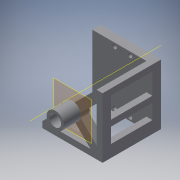
# Autodesk Inventor part: Sy_holder
Saved by Autodesk Inventor 2018 (Build 220112000, 112)
## iProperties
Created: 2018-10-01
Part Number: Sy_holder
Material: Generic
Document SubType Name: Modeling
Designer: David
Density: 1 g/cm^3
Appearance: Default
Author: David
Autodesk Inventor part; units mm, degrees
ref_plane "YZ Plane" through (0, 0, 0) normal (1, 0, 0) x (0, 1, 0)
ref_plane "XZ Plane" through (0, 0, 0) normal (0, 1, 0) x (-1, 0, 0)
ref_plane "XY Plane" through (0, 0, 0) normal (0, 0, 1) x (1, 0, 0)
sketch "Sketch1" plane through (0, 0, 0) normal (0, 1, 0) x (-1, 0, 0)
  line L0 (-17.5, -17.5) -> (17.5, -17.5)
  line L1 (17.5, -17.5) -> (17.5, 17.5)
  line L2 (17.5, 17.5) -> (-17.5, 17.5)
  line L3 (-17.5, 17.5) -> (-17.5, -17.5)
  line L4 (-17.5, -17.5) -> (17.5, 17.5) construction
  line L5 (17.5, -17.5) -> (-17.5, 17.5) construction
  point P0 (0, 0)
  dimension "d0" = 35
  dimension "d1" = 35
  constraints: 12 end point, 2 midpoint, 2 parallel, 1 horizontal, 1 perpendicular
  measures "d0" distance of L2.end L1.end
  measures "d1" distance of L1.end L0.end
extrude "Extrusion1" add sketch "Sketch1" along normal blind 5
sketch "Sketch2" plane through (0, 0, 0) normal (0, -1, 0) x (1, 0, 0)
  circle A0 centre (4.5, 15.5) radius 1.25 projected
  circle A1 centre (-4.5, 15.5) radius 1.25 projected
  circle A2 centre (4.5, -15.5) radius 1.25 projected
  circle A3 centre (-4.5, -15.5) radius 1.25 projected
  point P0 (0, 0)
extrude "Extrusion2" cut sketch "Sketch2" against normal blind 5
sketch "Sketch3" plane through (0, 0, 0) normal (0, -1, 0) x (1, 0, 0)
  line L0 (-17.5, -17.5) -> (-17.5, 17.5) projected
  line L1 (-17.5, -17.5) -> (-14, -17.5)
  line L2 (-14, -17.5) -> (-14, -14)
  line L3 (-14, -14) -> (-17.5, -14)
  line L4 (-17.5, -14) -> (-17.5, -17.5)
  line L5 (17.5, 17.5) -> (17.5, -17.5) projected
  line L6 (17.5, -17.5) -> (10.5, -17.5)
  line L7 (10.5, -17.5) -> (10.5, -14)
  line L8 (10.5, -14) -> (17.5, -14)
  line L9 (17.5, -14) -> (17.5, -17.5)
  line L10 (17.5, -14) -> (14, -14)
  line L11 (14, -14) -> (14, -10.5)
  line L12 (14, -10.5) -> (17.5, -10.5)
  line L13 (17.5, -10.5) -> (17.5, -14)
  line L14 (17.5, 17.5) -> (14, 17.5)
  line L15 (14, 17.5) -> (14, 14)
  line L16 (14, 14) -> (17.5, 14)
  line L17 (17.5, 14) -> (17.5, 17.5)
  line L18 (17.5, -17.5) -> (-17.5, -17.5) projected
  line L19 (1.75, -17.5) -> (-1.75, -17.5)
  line L20 (-1.75, -17.5) -> (-1.75, -14)
  line L21 (-1.75, -14) -> (1.75, -14)
  line L22 (1.75, -14) -> (1.75, -17.5)
  line L23 (17.5, 17.5) -> (17.5, -17.5) projected
  line L24 (17.5, 1.75) -> (14, 1.75)
  line L25 (14, 1.75) -> (14, -1.75)
  line L26 (14, -1.75) -> (17.5, -1.75)
  line L27 (17.5, -1.75) -> (17.5, 1.75)
  point P0 (0, 0)
  dimension "d6" = 3.5
  dimension "d7" = 3.5
  dimension "d8" = 7
  dimension "d9" = 3.5
  dimension "d10" = 3.5
  dimension "d11" = 3.5
  dimension "d12" = 3.5
  dimension "d13" = 3.5
  dimension "d14" = 3.5
  dimension "d15" = 3.5
  dimension "d16" = 3.5
  dimension "d17" = 3.5
  dimension "d18" = 1.75
  dimension "d19" = 1.75
  constraints: 48 end point, 12 parallel, 6 horizontal, 6 perpendicular, 2 point on line
  measures "d6" distance of L3.end L2.end
  measures "d7" distance of L2.end L1.end
  measures "d8" distance of L7.end L8.end
  measures "d9" distance of L6.end L7.end
  measures "d10" distance of L11.end L12.end
  measures "d11" distance of L10.end L11.end
  measures "d12" distance of L16.end L15.end
  measures "d13" distance of L15.end L14.end
  measures "d14" distance of L20.end L21.end
  measures "d15" distance of L19.end L20.end
  measures "d16" distance of L26.end L25.end
  measures "d17" distance of L25.end L24.end
  measures "d18" distance from line of point (0, 0) L22
  measures "d19" distance from line of point (0, 0) L26
extrude "Extrusion3" add sketch "Sketch3" along normal blind 24
sketch "Sketch4" plane through (0, -24, 0) normal (0, -1, 0) x (1, 0, 0)
  line L0 (-17.5, -14) -> (-14, -14) projected
  line L1 (14, 14) -> (14, 17.5) projected
  line L2 (10.5, -17.5) -> (10.5, -14) projected
  line L3 (14, -10.5) -> (17.5, -10.5) projected
  line L4 (-17.5, -14) -> (-17.5, -17.5) projected
  line L5 (-17.5, -14) -> (-17.5, -17.5)
  line L6 (17.5, 17.5) -> (17.5, -17.5) projected
  line L7 (-17.5, -17.5) -> (17.5, -17.5)
  line L8 (17.5, -17.5) -> (17.5, 17.5)
  line L9 (17.5, 17.5) -> (14, 17.5) projected
  line L10 (17.5, 17.5) -> (14, 17.5)
  line L11 (14, -14) -> (10.5, -14) projected
  line L12 (14, 17.5) -> (14, 14) projected
  line L13 (-17.5, -14) -> (-4.8221, -1.3221)
  line L14 (1.3221, 4.8221) -> (14, 17.5)
  line L15 (-10.5, -14) -> (-1.3221, -4.8221)
  line L16 (4.8221, 1.3221) -> (14, 10.5)
  line L17 (10.5, -14) -> (7.875, -11.375)
  line L18 (4.375, -7.875) -> (1.3221, -4.8221)
  line L19 (14, -10.5) -> (11.375, -7.875)
  line L20 (7.875, -4.375) -> (4.8221, -1.3221)
  line L21 (-10.5, -14) -> (-1.75, -14)
  line L22 (5.25, -14) -> (10.5, -14)
  circle A0 centre (0, 0) radius 3.415
  arc A1 (-1.3221, -4.8221) -> (1.3221, -4.8221) centre (0, 0) ccw
  arc A2 (4.8221, -1.3221) -> (4.8221, 1.3221) centre (0, 0) ccw
  arc A3 (1.3221, 4.8221) -> (-4.8221, -1.3221) centre (0, 0) ccw
  line L23 (10.5, -14) -> (7.875, -11.375)
  line L24 (10.5, -14) -> (14, -14) projected
  line L25 (5.25, -14) -> (10.5, -14)
  line L26 (-1.75, -17.5) -> (-1.75, -14) projected
  line L27 (-1.75, -14) -> (5.25, -14)
  line L28 (14, -1.75) -> (14, 1.75) projected
  line L29 (7.875, -4.375) -> (11.375, -7.875)
  line L30 (7.875, -11.375) -> (4.375, -7.875)
  line L31 (14, 10.5) -> (14, -10.5)
  point P0 (-14, -17.5)
  point P1 (17.5, 14)
  point P2 (17.5, -1.75)
  dimension "d28" = 6.83
  constraints: 40 end point, 6 point on circle, 5 parallel, 4 centre point, 3 horizontal, 3 perpendicular, 2 coincident, 2 collinear, 2 vertical, 1 point on line
  measures "d28" diameter of A0
ref_plane "Work Plane1" through (-3.5355, -24, 3.5355) normal (-0.7071068, 0, 0.7071068) x (0, -1, 0)
ref_plane "Work Plane2" through (0, -29, 0) normal (0, -1, 0) x (1, 0, 0)
sketch "Sketch6" plane through (0, -29, 0) normal (0, -1, 0) x (1, 0, 0)
  circle A0 centre (0, 0) radius 3.415
  circle A1 centre (0, 0) radius 5
  constraints: 2 centre point, 2 coincident
extrude "Extrusion6" add sketch "Sketch6" along normal blind 10
sketch "Sketch7" plane through (-3.5355, -24, 3.5355) normal (-0.7071068, 0, 0.7071068) x (0, -1, 0)
  circle A0 centre (8.733, 0) radius 1
  point P0 (-24, 0)
  dimension "d31" = 2
  constraints: 1 centre point
  measures "d31" diameter of A0
extrude "Extrusion7" cut sketch "Sketch7" against normal blind 2
extrude "Extrusion9" add sketch "Sketch4" along normal blind 5 contours L7 L26 L27 L22 L2 | L2 L17 L30 L18 A1 L15 L21 L26 L7 L4 L13 A3 L14 L9 L6
body "Solid1"
